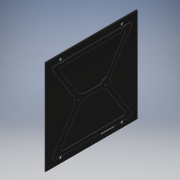
# Autodesk Inventor part: Structure_-X
Saved by Autodesk Inventor 2018 (Build 220112000, 112)
## iProperties
Created: 2018-07-04
Part Number: Structure_-X
Material: Aluminum 6061
Document SubType Name: Modeling
Designer: Bradley
Density: 2.7 g/cm^3
Appearance: Anodized - Dark Gray
Mass: 31.0491 g
Surface Area: 206.761 cm^2
Volume: 11.4997 cm^3
Author: Bradley
Autodesk Inventor part; units mm, degrees
ref_plane "YZ Plane" through (0, 0, 0) normal (1, 0, 0) x (0, 1, 0)
ref_plane "XZ Plane" through (0, 0, 0) normal (0, 1, 0) x (-1, 0, 0)
ref_plane "XY Plane" through (0, 0, 0) normal (0, 0, 1) x (1, 0, 0)
sketch "Sketch1" plane through (0, 0, 0) normal (1, 0, 0) x (0, 1, 0)
  line L0 (-48.5, -50) -> (48.5, -50)
  line L1 (48.5, -50) -> (48.5, 50)
  line L2 (48.5, 50) -> (-48.5, 50)
  line L3 (-48.5, 50) -> (-48.5, -50)
  line L4 (-48.5, -50) -> (48.5, 50) construction
  line L5 (48.5, -50) -> (-48.5, 50) construction
  point P0 (0, 0)
  dimension "d0" = 97
  dimension "d1" = 100
  constraints: 12 end point, 2 midpoint, 2 parallel, 1 horizontal, 1 perpendicular
  measures "d0" distance of L2.end L1.end
  measures "d1" distance of L1.end L0.end
extrude "Extrusion1" add sketch "Sketch1" along normal mid plane 1
sketch "Sketch2" plane through (0.5, 0, 0) normal (1, 0, 0) x (0, 0, -1)
  line L0 (45, -32.5) -> (-45, -32.5) construction
  line L1 (-45, -32.5) -> (-45, 32.5) construction
  line L2 (-45, 32.5) -> (45, 32.5) construction
  line L3 (45, 32.5) -> (45, -32.5) construction
  line L4 (45, -32.5) -> (-45, 32.5) construction
  line L5 (-45, -32.5) -> (45, 32.5) construction
  line L6 (0, -14) -> (0, 14) construction
  point P0 (0, 0)
  point P1 (0, 0)
  dimension "d5" = 90
  dimension "d6" = 65
  dimension "d14" = 28
  constraints: 14 end point, 6 coincident, 4 midpoint, 2 parallel, 1 horizontal, 1 perpendicular, 1 vertical
  measures "d5" distance of L1.end L2.end
  measures "d6" distance of L0.end L1.end
  measures "d14" distance of L6.start L6.end
hole "Hole1" at (0.5, -32.5, 45) at (0.5, 32.5, 45) at (0.5, 32.5, -45) at (0.5, -32.5, -45) at (0.5, -14, 0) at (0.5, 14, 0) direction (-1, 0, 0) diameter 3.2 end through all clearance for "Socket Head Cap Screw" size "M3" standard "Ansi Metric M Profile"
sketch "Sketch3" plane through (-0.5, 0, 0) normal (-1, 0, 0) x (0, 0, 1)
  circle A0 centre (0, -14) radius 1.6 projected
  circle A1 centre (-45, 32.5) radius 1.6 projected
  circle A2 centre (45, -32.5) radius 1.6 projected
  circle A3 centre (45, 32.5) radius 1.6 projected
  circle A4 centre (-45, -32.5) radius 1.6 projected
  circle A5 centre (0, 14) radius 1.6 projected
  line L0 (-50, 48.5) -> (-50, -48.5) projected
  line L1 (-50, -48.5) -> (50, -48.5) projected
  line L2 (50, -48.5) -> (50, 48.5) projected
  line L3 (50, 48.5) -> (-50, 48.5) projected
  circle A6 centre (0, 14) radius 4
  circle A7 centre (0, -14) radius 1.6 projected
  circle A8 centre (0, -14) radius 4
  point P0 (0, 0)
  dimension "d15" = 8
  constraints: 2 centre point, 2 coincident, 1 equal radius
  measures "d15" diameter of A6
extrude "Extrusion2" add sketch "Sketch3" along normal blind 3.25 contours A6 | A8
fillet "Fillet2" radius 0.381 2 edges at (-0.5, 14, -4) (-0.5, -14, -4)
chamfer "Chamfer1" distance 0.5 angle 45 2 edges at (-3.75, 14, -4) (-3.75, -14, -4)
sketch "Sketch4" plane through (0.5, 0, 0) normal (1, 0, 0) x (0, 0, -1)
  circle A0 centre (0, -14) radius 1.6 projected
  circle A1 centre (45, 32.5) radius 1.6 projected
  circle A2 centre (-45, -32.5) radius 1.6 projected
  circle A3 centre (-45, 32.5) radius 1.6 projected
  circle A4 centre (45, -32.5) radius 1.6 projected
  circle A5 centre (0, 14) radius 1.6 projected
  line L0 (50, -48.5) -> (50, 48.5) projected
  line L1 (50, 48.5) -> (-50, 48.5) projected
  line L2 (-50, 48.5) -> (-50, -48.5) projected
  line L3 (-50, -48.5) -> (50, -48.5) projected
  line L4 (-43, 41.4) -> (-39, 41.4)
  line L5 (-39, 41.4) -> (-39, -41.4)
  line L6 (-39, -41.4) -> (-43, -41.4)
  arc A6 (-43, -34.7361) -> (-43, -30.2639) centre (-45, -32.5) ccw
  arc A7 (-43, 30.2639) -> (-43, 34.7361) centre (-45, 32.5) ccw
  circle A8 centre (-45, 32.5) radius 1.6 projected
  line L7 (-43, -41.4) -> (-43, -34.7361)
  line L8 (-43, -30.2639) -> (-43, 30.2639)
  line L9 (-43, 34.7361) -> (-43, 41.4)
  line L10 (50, -48.5) -> (-50, -48.5) construction
  line L11 (0, -48.5) -> (0, 48.5) construction
  line L12 (43, 41.4) -> (39, 41.4)
  line L13 (39, 41.4) -> (39, -41.4)
  line L14 (39, -41.4) -> (43, -41.4)
  arc A9 (43, -30.2639) -> (43, -34.7361) centre (45, -32.5) ccw
  arc A10 (43, 34.7361) -> (43, 30.2639) centre (45, 32.5) ccw
  line L15 (43, -41.4) -> (43, -34.7361)
  line L16 (43, -30.2639) -> (43, 30.2639)
  line L17 (43, 34.7361) -> (43, 41.4)
  circle A11 centre (0, -14) radius 5
  circle A12 centre (0, 14) radius 5
  line L18 (-39, -41.4) -> (-2.7769, -18.158)
  line L19 (39, -41.4) -> (2.7769, -18.158)
  line L20 (39, 41.4) -> (2.7769, 18.158)
  line L21 (-39, 41.4) -> (-2.7769, 18.158)
  line L22 (-39, -36.6474) -> (-4.937, -14.7914)
  line L23 (-4.937, 14.7914) -> (-39, 36.6474)
  line L24 (4.937, 14.7914) -> (39, 36.6474)
  line L25 (4.937, -13.2086) -> (39, -35.0646)
  line L26 (2, -9.4174) -> (2, 9.4174)
  line L27 (-2, -9.4174) -> (-2, 9.4174)
  circle A13 centre (0, -14) radius 1.6 construction
  line L28 (0, -14) -> (-39, -39.0237) construction
  point P0 (0, -15)
  dimension "d23" = 3
  dimension "d24" = 86
  dimension "d25" = 82.8
  dimension "d26" = 4
  dimension "d32" = 10
  dimension "d33" = 4
  dimension "d34" = 4
  constraints: 48 end point, 20 point on circle, 10 symmetric about line, 8 equal length, 6 centre point, 6 parallel, 5 perpendicular, 5 point on line, 4 vertical, 2 coincident, 2 collinear, 2 concentric, 2 equal radius, 2 midpoint, 3 other
  measures "d23" radius of A6
  measures "d24" distance between parallel lines of L15 L7
  measures "d25" distance of L4.end L5.end
  measures "d26" distance between parallel lines of L5 L7
  measures "d32" diameter of A11
  measures "d33" distance between parallel lines of L18 L22
  measures "d34" distance between parallel lines of L26 L27
extrude "Extrusion4" add sketch "Sketch4" along normal blind 1 contours L4 L5 L6 L7 A6 L8 A7 L9 | L21 A12 L23 L5 | A12 | L22 A11 L18 L5 | L20 L13 L24 A12 | A11 | A12 L26 A11 L27 | L12 L17 A10 L16 A9 L15 L14 L13 | A11 L25 L13 L19
fillet "Fillet3" radius 2 28 edges at (1, -41.4, 39) (1, -36.6474, 39) (1, -30.2639, 43) (1, -34.7361, 43) (1, -18.158, 2.7769) (1, -18.158, -2.7769) (1, -13.2086, -4.937) (1, -9.4174, -2) (1, -9.4174, 2) (1, -14.7914, 4.937) (1, 34.7361, 43) (1, 30.2639, 43) (1, 36.6474, 39) (1, 41.4, 39) (1, 14.7914, 4.937) (1, 9.4174, 2) (1, 9.4174, -2) (1, 14.7914, -4.937) (1, 18.158, -2.7769) (1, 18.158, 2.7769) (1, 36.6474, -39) (1, 41.4, -39) (1, 34.7361, -43) (1, 30.2639, -43) (1, -30.2639, -43) (1, -34.7361, -43) (1, -41.4, -39) (1, -35.0646, -39)
fillet "Fillet3" radius 1 4 edges at (1, -41.4, -43) (1, 41.4, -43) (1, 41.4, 43) (1, -41.4, 43)
sketch "Sketch5" plane through (0.5, 0, 0) normal (1, 0, 0) x (0, 0, -1)
  line L0 (50, -48.5) -> (50, 48.5) projected
  line L1 (50, 48.5) -> (-50, 48.5) projected
  line L2 (-50, 48.5) -> (-50, -48.5) projected
  line L3 (-50, -48.5) -> (50, -48.5) projected
  circle A0 centre (45, -32.5) radius 1.6 projected
  circle A1 centre (-45, 32.5) radius 1.6 projected
  circle A2 centre (-45, -32.5) radius 1.6 projected
  circle A3 centre (45, 32.5) radius 1.6 projected
  arc A4 (-3.7548, 18.7855) -> (-1.9106, 18.6206) centre (-2.6748, 20.4688) ccw projected
  arc A5 (1.9106, 18.6206) -> (-1.9106, 18.6206) centre (0, 14) ccw projected
  arc A6 (1.9106, 18.6206) -> (3.7548, 18.7855) centre (2.6748, 20.4688) ccw projected
  line L4 (3.7548, 18.7855) -> (38.5064, 41.0833) projected
  arc A7 (39.5865, 41.4) -> (38.5064, 41.0833) centre (39.5865, 39.4) ccw projected
  line L5 (39.5865, 41.4) -> (42, 41.4) projected
  arc A8 (43, 40.4) -> (42, 41.4) centre (42, 40.4) ccw projected
  line L6 (43, 40.4) -> (43, 35.5) projected
  arc A9 (42.6, 34.3) -> (43, 35.5) centre (41, 35.5) ccw projected
  arc A10 (42.6, 34.3) -> (42.6, 30.7) centre (45, 32.5) ccw projected
  arc A11 (43, 29.5) -> (42.6, 30.7) centre (41, 29.5) ccw projected
  line L7 (43, 29.5) -> (43, -29.5) projected
  arc A12 (42.6, -30.7) -> (43, -29.5) centre (41, -29.5) ccw projected
  arc A13 (42.6, -30.7) -> (42.6, -34.3) centre (45, -32.5) ccw projected
  arc A14 (43, -35.5) -> (42.6, -34.3) centre (41, -35.5) ccw projected
  line L8 (43, -35.5) -> (43, -40.4) projected
  arc A15 (42, -41.4) -> (43, -40.4) centre (42, -40.4) ccw projected
  line L9 (42, -41.4) -> (39.5865, -41.4) projected
  arc A16 (38.5064, -41.0833) -> (39.5865, -41.4) centre (39.5865, -39.4) ccw projected
  line L10 (38.5064, -41.0833) -> (3.7548, -18.7855) projected
  arc A17 (3.7548, -18.7855) -> (1.9106, -18.6206) centre (2.6748, -20.4688) ccw projected
  arc A18 (-1.9106, -18.6206) -> (1.9106, -18.6206) centre (0, -14) ccw projected
  arc A19 (-1.9106, -18.6206) -> (-3.7548, -18.7855) centre (-2.6748, -20.4688) ccw projected
  line L11 (-3.7548, -18.7855) -> (-38.5064, -41.0833) projected
  arc A20 (-39.5865, -41.4) -> (-38.5064, -41.0833) centre (-39.5865, -39.4) ccw projected
  line L12 (-39.5865, -41.4) -> (-42, -41.4) projected
  arc A21 (-43, -40.4) -> (-42, -41.4) centre (-42, -40.4) ccw projected
  line L13 (-43, -40.4) -> (-43, -35.5) projected
  arc A22 (-42.6, -34.3) -> (-43, -35.5) centre (-41, -35.5) ccw projected
  arc A23 (-42.6, -34.3) -> (-42.6, -30.7) centre (-45, -32.5) ccw projected
  arc A24 (-43, -29.5) -> (-42.6, -30.7) centre (-41, -29.5) ccw projected
  line L14 (-43, -29.5) -> (-43, 29.5) projected
  arc A25 (-42.6, 30.7) -> (-43, 29.5) centre (-41, 29.5) ccw projected
  arc A26 (-42.6, 30.7) -> (-42.6, 34.3) centre (-45, 32.5) ccw projected
  arc A27 (-43, 35.5) -> (-42.6, 34.3) centre (-41, 35.5) ccw projected
  line L15 (-43, 35.5) -> (-43, 40.4) projected
  arc A28 (-42, 41.4) -> (-43, 40.4) centre (-42, 40.4) ccw projected
  line L16 (-42, 41.4) -> (-39.5865, 41.4) projected
  arc A29 (-38.5064, 41.0833) -> (-39.5865, 41.4) centre (-39.5865, 39.4) ccw projected
  line L17 (-38.5064, 41.0833) -> (-3.7548, 18.7855) projected
  line L18 (43, -29.5) -> (43, 29.5) projected
  line L19 (44, 10) -> (44.5, 10)
  line L20 (45.5, 11) -> (45.5, 24)
  line L21 (44.5, 25) -> (44, 25)
  line L22 (43, 24) -> (43, 11)
  arc A30 (44.5, 10) -> (45.5, 11) centre (44.5, 11) ccw
  arc A31 (45.5, 24) -> (44.5, 25) centre (44.5, 24) ccw
  arc A32 (44, 25) -> (43, 24) centre (44, 24) ccw
  arc A33 (43, 11) -> (44, 10) centre (44, 11) ccw
  point P0 (0, 0)
  point P1 (43, 10)
  point P2 (45.5, 25)
  point P3 (45.5, 10)
  point P4 (43, 25)
  dimension "d39" = 2.5
  dimension "d40" = 15
  dimension "d41" = 10
  dimension "d42" = 1
  constraints: 9 point on line, 8 end point, 8 point on circle, 8 tangent, 4 centre point, 3 equal radius, 2 parallel, 1 horizontal, 1 perpendicular
  measures "d39" distance of point (43, 25) point (45.5, 25)
  measures "d40" distance of point (45.5, 10) point (45.5, 25)
  measures "d41" distance from line of L19 point (0, 0)
  measures "d42" radius of A30
extrude "Extrusion5" cut sketch "Sketch5" against normal through all contours A32 L21 A31 L20 A30 L19 A33 L7
chamfer "Chamfer2" distance 0.25 angle 45 8 edges at (-0.5, 24.7071, -43.2929) (-0.5, 17.5, -43) (-0.5, 10.2929, -43.2929) (-0.5, 10, -44.25) (-0.5, 10.2929, -45.2071) (-0.5, 17.5, -45.5) (-0.5, 24.7071, -45.2071) (-0.5, 25, -44.25)
equation "\"d33\" = d26"
equation "\"d34\" = d26"
body "Solid1"
